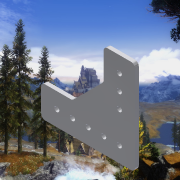
# Autodesk Inventor part: C21_TK_TriangleGusset
Saved by Autodesk Inventor 2015 SP1 (Build 190203100, 203)
## iProperties
Created: 2016-01-26
Part Number: C21_TK_TriangleGusset
Material: Aluminum 6061
Document SubType Name: Modeling
Designer: TheeTimatahee
Density: 2.7 g/cm^3
Appearance: Aluminum - Flat
Mass: 29.4062 g
Surface Area: 80.8896 cm^2
Volume: 10.8912 cm^3
Author: TheeTimatahee
Autodesk Inventor part; units mm, degrees
ref_plane "YZ Plane" through (0, 0, 0) normal (1, 0, 0) x (0, 1, 0)
ref_plane "XZ Plane" through (0, 0, 0) normal (0, 1, 0) x (-1, 0, 0)
ref_plane "XY Plane" through (0, 0, 0) normal (0, 0, 1) x (1, 0, 0)
sketch "Sketch1" plane through (0, 0, 0) normal (0, 0, 1) x (1, 0, 0)
  line L0 (-32.8613, -32.8613) -> (43.3387, -32.8613)
  line L1 (43.3387, -32.8613) -> (43.3387, 43.3387)
  line L2 (-32.8613, -32.8613) -> (43.3387, 43.3387) construction
  line L3 (43.3387, 43.3387) -> (-32.8613, -32.8613)
  line L4 (43.3387, 43.3387) -> (17.9387, 43.3387)
  line L5 (17.9387, 43.3387) -> (17.9387, 17.9387)
  line L6 (43.3387, 22.2601) -> (43.3387, 43.3387)
  line L7 (-32.8613, -32.8613) -> (-7.4613, -32.8613)
  line L8 (-7.4613, -32.8613) -> (-7.4613, -7.4613)
  line L9 (-7.4613, -7.4613) -> (-32.8613, -7.4613)
  line L10 (-32.8613, -7.4613) -> (-32.8613, -32.8613)
  point P0 (0, 0)
  dimension "d1" = 76.2
  dimension "d2" = 76.2
  dimension "d7" = 25.4
  dimension "d8" = 25.4
  constraints: 22 end point, 3 horizontal, 3 parallel, 3 perpendicular, 3 point on line, 1 collinear
  measures "d1" distance of L0.start L0.end
  measures "d2" distance of L0.end L1.end
  measures "d7" distance of L1.end L4.end
  measures "d8" distance of L8.end L9.end
extrude "Extrusion1" add sketch "Sketch1" along normal blind 3.175
fillet "Fillet2" radius 3.175 7 edges at (17.9387, 43.3387, 1.5875) (43.3387, 43.3387, 1.5875) (17.9387, 17.9387, 1.5875) (-7.4613, -7.4613, 1.5875) (-32.8613, -7.4613, 1.5875) (-32.8613, -32.8613, 1.5875) (43.3387, -32.8613, 1.5875)
sketch "Sketch2" plane through (0, 0, 3.175) normal (0, 0, 1) x (1, 0, 0)
  arc A0 (20.0074, -20.0851) -> (15.8701, -20.0851) centre (17.9387, -20.1613) ccw projected
  line L0 (20.0074, -20.0851) -> (28.5701, -20.0851) projected
  arc A1 (32.7074, -20.0851) -> (28.5701, -20.0851) centre (30.6387, -20.1613) ccw projected
  line L1 (32.7074, -20.0851) -> (43.3387, -20.0851) projected
  line L2 (43.3387, -20.0851) -> (43.3387, -7.4613) projected
  line L3 (-693.2613, -7.4613) -> (43.3387, -7.4613) projected
  line L4 (-693.2613, -7.4613) -> (-693.2613, -20.0851) projected
  line L5 (-693.2613, -20.0851) -> (-682.6299, -20.0851) projected
  arc A2 (-678.4926, -20.0851) -> (-682.6299, -20.0851) centre (-680.5613, -20.1613) ccw projected
  line L6 (-678.4926, -20.0851) -> (-669.9299, -20.0851) projected
  arc A3 (-665.7926, -20.0851) -> (-669.9299, -20.0851) centre (-667.8613, -20.1613) ccw projected
  line L7 (-665.7926, -20.0851) -> (-657.2299, -20.0851) projected
  arc A4 (-653.0926, -20.0851) -> (-657.2299, -20.0851) centre (-655.1613, -20.1613) ccw projected
  line L8 (-653.0926, -20.0851) -> (-644.5299, -20.0851) projected
  arc A5 (-640.3926, -20.0851) -> (-644.5299, -20.0851) centre (-642.4613, -20.1613) ccw projected
  line L9 (-640.3926, -20.0851) -> (-631.8299, -20.0851) projected
  arc A6 (-627.6926, -20.0851) -> (-631.8299, -20.0851) centre (-629.7613, -20.1613) ccw projected
  line L10 (-627.6926, -20.0851) -> (-272.9448, -20.0851) projected
  arc A7 (-242.32, -20.0851) -> (-272.9448, -20.0851) centre (-257.6324, -29.1216) ccw projected
  line L11 (-242.32, -20.0851) -> (-22.2299, -20.0851) projected
  arc A8 (-18.0926, -20.0851) -> (-22.2299, -20.0851) centre (-20.1613, -20.1613) ccw projected
  line L12 (-18.0926, -20.0851) -> (-9.5299, -20.0851) projected
  arc A9 (-5.3926, -20.0851) -> (-9.5299, -20.0851) centre (-7.4613, -20.1613) ccw projected
  line L13 (-5.3926, -20.0851) -> (3.1701, -20.0851) projected
  arc A10 (7.3074, -20.0851) -> (3.1701, -20.0851) centre (5.2387, -20.1613) ccw projected
  line L14 (7.3074, -20.0851) -> (15.8701, -20.0851) projected
  arc A11 (-84.7976, -15.8974) -> (-84.7976, -10.792) centre (-84.7976, -13.3447) ccw projected
  line L15 (-84.7976, -15.8974) -> (-94.3226, -15.8974) projected
  arc A12 (-94.3226, -10.792) -> (-94.3226, -15.8974) centre (-94.3226, -13.3447) ccw projected
  line L16 (-94.3226, -10.792) -> (-84.7976, -10.792) projected
  arc A13 (-604.3151, -10.792) -> (-604.3151, -15.8974) centre (-604.3151, -13.3447) ccw projected
  line L17 (-604.3151, -10.792) -> (-594.7901, -10.792) projected
  arc A14 (-594.7901, -15.8974) -> (-594.7901, -10.792) centre (-594.7901, -13.3447) ccw projected
  line L18 (-594.7901, -15.8974) -> (-604.3151, -15.8974) projected
  arc A15 (-564.9959, -10.792) -> (-564.9959, -15.8974) centre (-564.9959, -13.3447) ccw projected
  line L19 (-564.9959, -10.792) -> (-555.4709, -10.792) projected
  arc A16 (-555.4709, -15.8974) -> (-555.4709, -10.792) centre (-555.4709, -13.3447) ccw projected
  line L20 (-555.4709, -15.8974) -> (-564.9959, -15.8974) projected
  arc A17 (-55.0034, -10.792) -> (-55.0034, -15.8974) centre (-55.0034, -13.3447) ccw projected
  line L21 (-55.0034, -10.792) -> (-45.4784, -10.792) projected
  arc A18 (-45.4784, -15.8974) -> (-45.4784, -10.792) centre (-45.4784, -13.3447) ccw projected
  line L22 (-45.4784, -15.8974) -> (-55.0034, -15.8974) projected
  arc A19 (30.7149, 28.5701) -> (30.7149, 32.7074) centre (30.6387, 30.6387) ccw projected
  line L23 (30.7149, 20.0074) -> (30.7149, 28.5701) projected
  arc A20 (30.7149, 15.8701) -> (30.7149, 20.0074) centre (30.6387, 17.9387) ccw projected
  line L24 (30.7149, 7.3074) -> (30.7149, 15.8701) projected
  arc A21 (30.7149, 3.1701) -> (30.7149, 7.3074) centre (30.6387, 5.2387) ccw projected
  line L25 (30.7149, -7.4613) -> (30.7149, 3.1701) projected
  line L26 (43.3387, -7.4613) -> (30.7149, -7.4613) projected
  line L27 (43.3387, 221.1387) -> (43.3387, -7.4613) projected
  line L28 (43.3387, 221.1387) -> (30.7149, 221.1387) projected
  line L29 (30.7149, 190.6448) -> (30.7149, 221.1387) projected
  arc A22 (30.7149, 183.509) -> (30.7149, 190.6448) centre (30.6387, 187.0769) ccw projected
  line L30 (30.7149, 32.7074) -> (30.7149, 183.509) projected
  point P0 (0, 0)
  point P1 (30.6387, 5.2387)
  point P2 (30.6387, 30.6387)
hole "Hole1" at (30.6387, 30.6387, 3.175) at (30.6387, 5.2387, 3.175) at (30.6387, -20.1613, 3.175) at (5.2387, -20.1613, 3.175) at (-20.1613, -20.1613, 3.175) at (-7.4613, -20.1613, 3.175) at (17.9387, -20.1613, 3.175) at (30.6387, 17.9387, 3.175) direction (0, 0, -1) diameter 4.1402 end through all
body "Solid1"
